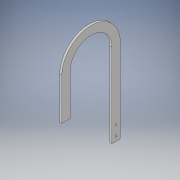
# Autodesk Inventor part: Hook Plate
Saved by Autodesk Inventor 2019.4 (Build 234330000, 330)
## iProperties
Created: 2020-03-10
Part Number: Hook Plate
Material: Generic
Document SubType Name: Modeling
Designer: admin
Density: 1 g/cm^3
Appearance: Default
Author: admin
Autodesk Inventor part; units mm, degrees
ref_plane "YZ Plane" through (0, 0, 0) normal (1, 0, 0) x (0, 1, 0)
ref_plane "XZ Plane" through (0, 0, 0) normal (0, 1, 0) x (-1, 0, 0)
ref_plane "XY Plane" through (0, 0, 0) normal (0, 0, 1) x (1, 0, 0)
sketch "Sketch1" plane through (0, 0, 0) normal (1, 0, 0) x (0, 1, 0)
  line L0 (0, 0) -> (200, 0)
  line L1 (0, 0) -> (0, 20)
  line L2 (0, 20) -> (200, 20)
  arc A0 (200, 20) -> (201.6312, 119.9734) centre (200, 70) ccw
  arc A1 (200, 0) -> (202.1069, 139.9683) centre (200, 70) ccw
  line L3 (201.6312, 119.9734) -> (102.1069, 119.9734)
  line L4 (102.1069, 119.9734) -> (102.1069, 139.9683)
  line L5 (102.1069, 139.9683) -> (202.1069, 139.9683)
  circle A2 centre (11.0857, 10) radius 2.2
  circle A3 centre (34.5336, 10) radius 2.2
  dimension "d0" = 20
  dimension "d1" = 200
  dimension "d2" = 200
  dimension "d3" = 100
  dimension "d4" = 50
  dimension "d5" = 4.4
  dimension "d6" = 4.4
  constraints: 12 end point, 4 centre point, 4 point on circle, 3 perpendicular, 2 horizontal, 1 coincident, 1 tangent, 1 vertical
  measures "d0" distance of L0.start L1.end
  measures "d1" distance of L1.end L2.end
  measures "d2" distance of L0.start L0.end
  measures "d3" distance of L4.end L5.end
  measures "d4" radius of A0
  measures "d5" diameter of A2
  measures "d6" diameter of A3
extrude "Extrusion1" add sketch "Sketch1" along normal blind 5
body "Solid1"
